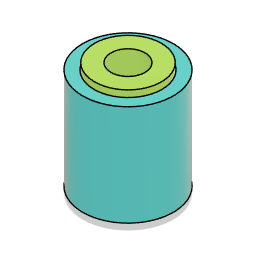
Mini_Barrett_Hand_ver2 (Autodesk Fusion 360 archive; units mm, degrees)
design "bush"
Autodesk Fusion 360 part; units mm, degrees
sketch "Sketch1" plane through (0, 0, 0) normal (0, 1, 0) x (1, 0, 0) in component "outer"
  circle A0 centre (0, 0) radius 4
  dimension "d1" = 8
  constraint coincident A0.centre origin
  measures "d1" diameter of A0
extrude "Extrude1" add sketch "Sketch1" along normal blind 8.9 makes body 1 in component "outer"
sketch "Sketch2" plane through (0, 0, 0) normal (0, -1, 0) x (1, 0, 0) in component "outer"
  circle A0 centre (0, 0) radius 4
  circle A1 centre (0, 0) radius 3
  dimension "d4" = 6
  constraint concentric A0 A1
  measures "d4" diameter of A1
extrude "Extrude2" cut sketch "Sketch2" against normal blind 12 contours A1 bodies 1 in component "outer"
sketch "Sketch1 (2)" plane through (0, 0, 0) normal (0, 1, 0) x (1, 0, 0) in component "inner"
  circle A0 centre (0, 0) radius 2.95
  dimension "d7" = 5.9
  constraint coincident A0.centre origin
  measures "d7" diameter of A0
extrude "Extrude1'" add sketch "Sketch1 (2)" along normal blind 10 separate body makes body 2 in component "inner"
sketch "Sketch2 (2)" plane through (0, 10, 0) normal (0, 1, 0) x (-1, 0, 0) in component "inner"
  circle A0 centre (0, 0) radius 2.95
  circle A1 centre (0, 0) radius 1.5
  dimension "d10" = 3
  constraint concentric A0 A1
  measures "d10" diameter of A1
extrude "Extrude2'" cut sketch "Sketch2 (2)" against normal blind 11 contours A1 bodies 2 in component "inner"
component "outer" placed x (1, 0, 0) y (0, 1, 0) z (0, 0, 1) at (0, 0, 0)
component "inner" placed x (1, 0, 0) y (0, 1, 0) z (0, 0, 1) at (0, -0.55, 0)
